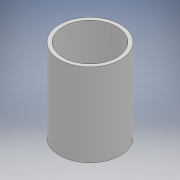
# Autodesk Inventor part: Black part to elbow
Saved by Autodesk Inventor 2017 (Build 210142000, 142)
## iProperties
Created: 2017-11-14
Part Number: Black part to elbow
Material: Generic
Document SubType Name: Modeling
Designer: DesignPC02
Density: 1 g/cm^3
Appearance: Default
Author: DesignPC02
Autodesk Inventor part; units mm, degrees
ref_plane "YZ Plane" through (0, 0, 0) normal (1, 0, 0) x (0, 1, 0)
ref_plane "XZ Plane" through (0, 0, 0) normal (0, 1, 0) x (-1, 0, 0)
ref_plane "XY Plane" through (0, 0, 0) normal (0, 0, 1) x (1, 0, 0)
sketch "Sketch2" plane through (0, 0, 0) normal (0, 0, 1) x (1, 0, 0)
  circle A0 centre (0, 0) radius 11
  circle A1 centre (0, 0) radius 9.7
  dimension "d5" = 22
  dimension "d7" = 1.3
  constraints: 2 centre point, 1 coincident
  measures "d5" diameter of A0
  measures "d7" radial gap between concentric circles of A0 A1
extrude "Extrusion2" add sketch "Sketch2" along normal mid plane 30
body "Solid2"
